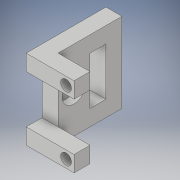
# Autodesk Inventor part: TensionerPlate
Saved by Autodesk Inventor 2017 (Build 210142000, 142)
## iProperties
Created: 2017-07-29
Part Number: TensionerPlate
Material: Generic
Document SubType Name: Modeling
Designer: User
Density: 1 g/cm^3
Appearance: Default
Author: User
Autodesk Inventor part; units mm, degrees
ref_plane "YZ Plane" through (0, 0, 0) normal (1, 0, 0) x (0, 1, 0)
ref_plane "XZ Plane" through (0, 0, 0) normal (0, 1, 0) x (-1, 0, 0)
ref_plane "XY Plane" through (0, 0, 0) normal (0, 0, 1) x (1, 0, 0)
sketch "Sketch1" plane through (0, 0, 0) normal (1, 0, 0) x (0, 1, 0)
  line L0 (31.75, 0) -> (31.75, -31.75)
  line L1 (31.75, -31.75) -> (0, -31.75)
  line L2 (0, -31.75) -> (0, 0)
  line L3 (25.4, 0) -> (25.4, -6.35)
  line L4 (25.4, -6.35) -> (6.35, -6.35)
  line L5 (6.35, -6.35) -> (6.35, 0)
  line L6 (6.35, -31.75) -> (25.4, -31.75)
  line L7 (0, 0) -> (6.35, 0)
  line L8 (25.4, 0) -> (31.75, 0)
  line L9 (6.35, -19.05) -> (25.4, -19.05)
  line L10 (25.4, -19.05) -> (25.4, -25.4)
  line L11 (25.4, -25.4) -> (6.35, -25.4)
  line L12 (6.35, -25.4) -> (6.35, -19.05)
  dimension "d6" = 6.35
  dimension "d8" = 19.05
  dimension "d9" = 6.35
  dimension "d10" = 6.35
  dimension "d11" = 6.35
  dimension "d19" = 31.75
  dimension "d20" = 31.75
  constraints: 26 end point, 6 parallel, 4 horizontal, 3 perpendicular, 1 point on line
  measures "d6" distance between parallel lines of L2 L5
  measures "d8" distance of L10.end L11.end
  measures "d9" distance of L9.end L10.end
  measures "d10" distance between parallel lines of L1 L11
  measures "d11" distance between parallel lines of L2 L12
  measures "d19" distance of L0.start L0.end
  measures "d20" distance of L1.end L2.end
extrude "Extrusion1" add sketch "Sketch1" along normal blind 6.35
sketch "Sketch2" plane through (6.35, 0, 0) normal (1, 0, 0) x (0, 0, -1)
  line L0 (19.05, 25.4) -> (25.4, 25.4) projected
  line L1 (25.4, 25.4) -> (25.4, 6.35) projected
  line L2 (25.4, 6.35) -> (19.05, 6.35) projected
  line L3 (19.05, 6.35) -> (19.05, 25.4) projected
  line L4 (0, 0) -> (31.75, 0) projected
  line L5 (31.75, 0) -> (31.75, 31.75) projected
  line L6 (31.75, 31.75) -> (0, 31.75) projected
  line L7 (0, 31.75) -> (0, 25.4) projected
  line L8 (0, 25.4) -> (6.35, 25.4) projected
  line L9 (6.35, 25.4) -> (6.35, 6.35) projected
  line L10 (6.35, 6.35) -> (0, 6.35) projected
  line L11 (0, 6.35) -> (0, 0) projected
  circle A0 centre (12.7, 15.875) radius 4.7625
  dimension "d14" = 9.525
  dimension "d15" = 15.875
  dimension "d16" = 6.35
  constraints: 1 centre point
  measures "d14" diameter of A0
  measures "d15" distance from line of L6 A0.centre
  measures "d16" distance from line of L9 A0.centre
extrude "Extrusion2" cut sketch "Sketch2" against normal blind 3.175 contours A0
sketch "Sketch3" plane through (0, 25.4, 0) normal (0, 0, 1) x (1, 0, 0)
  line L0 (0, 6.35) -> (0, 0) projected
  line L1 (0, 0) -> (6.35, 0) projected
  line L2 (6.35, 6.35) -> (6.35, 0) projected
  line L3 (0, 6.35) -> (6.35, 6.35) projected
  line L4 (0, -19.05) -> (0, -25.4) projected
  line L5 (0, -25.4) -> (6.35, -25.4) projected
  line L6 (6.35, -19.05) -> (6.35, -25.4) projected
  line L7 (0, -19.05) -> (6.35, -19.05) projected
  line L8 (0, 6.35) -> (19.05, 6.35)
  line L9 (19.05, 6.35) -> (19.05, 0)
  line L10 (19.05, 0) -> (0, 0)
  line L11 (0, 0) -> (0, 6.35)
  line L12 (0, -25.4) -> (19.05, -25.4)
  line L13 (19.05, -25.4) -> (19.05, -19.05)
  line L14 (19.05, -19.05) -> (0, -19.05)
  line L15 (0, -19.05) -> (0, -25.4)
  circle A0 centre (15.875, 3.175) radius 2.159
  circle A1 centre (15.875, -22.225) radius 2.159
  dimension "d21" = 19.05
  dimension "d22" = 4.318
  dimension "d23" = 3.175
  dimension "d24" = 4.318
  constraints: 16 end point, 4 parallel, 2 centre point, 2 horizontal, 2 perpendicular, 1 point on line
  measures "d21" distance of L9.end L10.end
  measures "d22" diameter of A0
  measures "d23" distance from line of L9 A0.centre
  measures "d24" diameter of A1
extrude "Extrusion3" add sketch "Sketch3" against normal blind 6.35 contours L8 L9 L10 L2 | L14 L13 L12 L6
equation "\"d20\" = d19"
body "Solid1"
